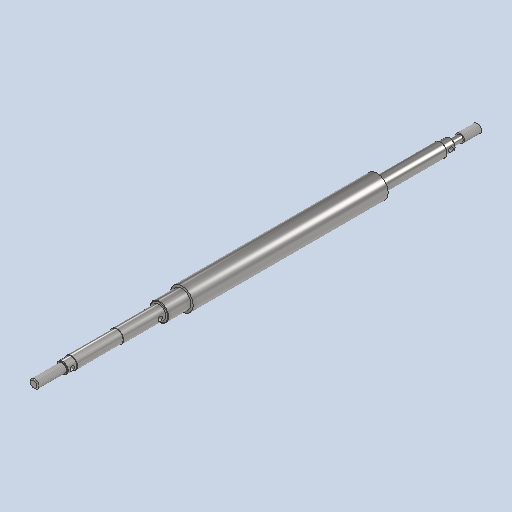
# Autodesk Inventor part: essieu arriere
Saved by Autodesk Inventor 2024 (Build 280153000, 153)
## iProperties
Created: 2022-10-04
Part Number: essieu arriere
Material: Acier inoxydable
Document SubType Name: Modeling
Designer: ropertth
Density: 8 g/cm^3
Appearance: Semi-poli
Mass: 74.8661 g
Surface Area: 48.0695 cm^2
Volume: 9.35827 cm^3
Author: ropertth
Autodesk Inventor part; units mm, degrees
ref_plane "YZ Plane" through (0, 0, 0) normal (1, 0, 0) x (0, 1, 0)
sketch "Esquisse1" plane through (0, 0, 0) normal (1, 0, 0) x (0, 1, 0)
  line L0 (5, -65) -> (5, -150.6)
  line L1 (5, -150.6) -> (2.9605, -150.6)
  line L2 (2.9605, -150.6) -> (2.9605, -178.6)
  line L3 (2.9605, -178.6) -> (1.919, -178.6)
  line L4 (1.919, -178.6) -> (1.919, -195.1)
  line L5 (1.919, -195.1) -> (0, -195.1)
  line L6 (4, -55) -> (2.9605, -55)
  line L7 (2.9605, -55) -> (2.9605, -36.5)
  line L8 (2.783, -16.5) -> (1.919, -16.5)
  line L9 (1.919, -16.5) -> (1.919, 0)
  line L10 (1.919, 0) -> (0, 0)
  line L11 (0, -195.1) -> (0, 0)
  line L12 (4, -55) -> (4, -65)
  line L13 (4, -65) -> (5, -65)
  line L14 (1.919, -16.5) -> (1.45, -16.5)
  line L15 (1.45, -16.5) -> (1.45, -8)
  line L16 (1.45, -8) -> (2, -8)
  line L17 (1.919, -12.5) -> (1.919, -16.5)
  line L18 (1.919, -178.6) -> (1.45, -178.6)
  line L19 (1.45, -178.6) -> (1.45, -187.1)
  line L20 (1.45, -187.1) -> (1.919, -187.1)
  line L21 (1.919, -187.1) -> (1.919, -178.6)
  line L22 (2.5, -16.5) -> (1.919, -16.5)
  line L23 (1.45, -12.5) -> (2.5, -12.5)
  line L24 (2.5, -12.5) -> (2.5, -16.5)
  line L25 (2.5, -178.6) -> (1.919, -178.6)
  line L26 (1.919, -178.6) -> (1.919, -182.6)
  line L27 (1.45, -182.6) -> (2.5, -182.6)
  line L28 (2.5, -182.6) -> (2.5, -178.6)
  line L29 (2.783, -16.5) -> (2.5, -16.5)
  line L30 (2.783, -16.5) -> (2.783, -36.5)
  line L31 (2.783, -36.5) -> (2.9605, -36.5)
  point P0 (1.919, -8)
  point P1 (1.919, -187.1)
  point P2 (2.4398, -178.6)
  point P3 (2.7415, -36.5)
  point P4 (2.7415, -16.5)
  dimension "d2" = 28
  dimension "d4" = 16.5
  dimension "d5" = 16.5
  dimension "d15" = 95.6
  dimension "d16" = 10
  dimension "d18" = 8.5
  dimension "d19" = 2.9
  dimension "d20" = 8.5
  dimension "d21" = 8
  dimension "d22" = 10
  dimension "d24" = 4
  dimension "d25" = 4
  dimension "d26" = 5
  dimension "d27" = 4
  dimension "d28" = 5
  dimension "d41" = 6
  constraints: 65 end point, 13 perpendicular, 9 point on line, 7 parallel, 6 horizontal, 2 collinear, 2 vertical, 1 midpoint
  measures "d2" distance of L1.end L2.end
  measures "d4" distance of L8.end L9.end
  measures "d5" distance of L3.end L4.end
  measures "d15" vertical distance of L0.end L6.end
  measures "d16" distance of L6.start L12.end
  measures "d18" distance of L14.end L15.end
  measures "d19" diameter of L15 L11
  measures "d20" distance of L18.end L19.end
  measures "d21" diameter of L12 L11
  measures "d22" diameter of L0 L11
  measures "d25" distance of L23.end L22.start
  measures "d26" diameter of L24 L11
  measures "d27" distance from line of point (2.44, -178.6) L27
  measures "d28" diameter of L28 L11
revolve "Révolution1" add sketch "Esquisse1" angle 360 about axis through (0, 0, -195.1) along (0, 0, 1) contours L0 L1 L2 L3 L18 L19 L20 L4 L5 L11 L10 L9 L16 L15 L14 L8 L30 L31 L7 L6 L12 L13 | L28 L27 L4 L3 | L4 L27 L19 L18 | L8 L9 L23 L24 | L14 L15 L23 L9 | L23 L15 L16 L9
fillet "Congé1" radius 0.5 2 edges at (0, -1.919, 0) (0, -1.919, -195.1)
thread "Filetage1" size "M4x0.7" class "6g" standard "ANSI Metric M Profile" full length
fillet "Congé2" radius 0.2 4 edges at (0, -2.5, -182.6) (0, -2.9605, -178.6) (0, -4, -55) (0, -2.5, -12.5)
sketch "Esquisse2" plane through (0, 0, -195.1) normal (0, 0, -1) x (-1, 0, 0)
  point P0 (0, 0)
  point P1 (0, 0)
  constraints: 1 coincident
hole "Perçage1" at (0, 0, -195.1) direction (0, 0, 1) diameter 1 depth 3 tip angle 118 countersink diameter 2 countersink angle 60
sketch "Esquisse3" plane through (0, 0, 0) normal (0, 0, 1) x (1, 0, 0)
  line L0 (0, 0) -> (-2.5, 0) construction
  circle A0 centre (0, 0) radius 2.5 construction
  circle A1 centre (0, 0) radius 2.5 construction
  line L1 (0, 0) -> (-5.0002, 0) construction
  circle A2 centre (0, 0) radius 2.9605 construction
  circle A3 centre (0, 0) radius 2.9605 construction
  point P0 (-2.9605, 0)
  constraints: 4 end point, 2 horizontal, 2 horizontal alignment, 1 coincident, 1 point on line, 2 other
ref_plane "Plan de construction1" through (-2.5, 0, 0) normal (-1, 0, 0) x (0, -1, 0)
sketch "Esquisse4" plane through (-2.5, 0, 0) normal (-1, 0, 0) x (0, -1, 0)
  line L0 (-4.9491, -12.5) -> (5.1773, -12.5)
  line L1 (5.1773, -12.5) -> (5.1773, -16.5)
  line L2 (5.1773, -16.5) -> (-4.9491, -16.5)
  line L3 (-4.9491, -16.5) -> (-4.9491, -12.5)
  line L4 (2.3, -182.6) -> (-2.3, -182.6) projected
  line L5 (2.7605, -178.6) -> (-2.7605, -178.6) projected
  line L6 (-3.4203, -182.6) -> (3.9321, -182.6)
  line L7 (3.9321, -182.6) -> (3.9321, -178.6)
  line L8 (3.9321, -178.6) -> (-3.4203, -178.6)
  line L9 (-3.4203, -178.6) -> (-3.4203, -182.6)
  point P0 (0, 0)
  constraints: 16 end point, 4 parallel, 2 horizontal, 2 perpendicular, 1 point on line
extrude "Extrusion1" cut sketch "Esquisse4" against normal blind 0.3
sketch "Esquisse6" plane through (-2.2, 0, 0) normal (-1, 0, 0) x (0, 0, 1)
  line L0 (0, 0) -> (-16.5, 0) construction
  line L1 (-16.5, 2.5) -> (-16.5, -2.5) construction
  line L2 (-12.5, 2.3) -> (-12.5, -2.3) construction
  line L3 (-178.6, -2.7605) -> (-178.6, 2.7605) projected
  line L4 (-182.6, -0.6708) -> (-182.6, 0.6708) projected
  point P0 (-14.5, 0)
  point P1 (-16.5, 1.1874)
  point P2 (-16.5, -1.1874)
  point P3 (-12.5, 0.6708)
  point P4 (-12.5, -0.6708)
  point P5 (-180.6, 0)
  dimension "d51" = 4
  dimension "d52" = 2
  dimension "d71" = 4
  dimension "d72" = 2
  constraints: 2 end point, 1 midpoint, 1 point on line
  measures "d51" distance between parallel lines of L1 L2
  measures "d52" distance from line of L2 point (-14.5, 0)
  measures "d71" distance between parallel lines of L3 L4
  measures "d72" distance from line of L3 point (-180.6, 0)
hole "Perçage2" at (-2.2, 0, -14.5) at (-2.2, 0, -180.6) direction (1, 0, 0) diameter 2 end through all
ref_plane "Plan de construction2" through (-2.9605, 0, 0) normal (-1, 0, 0) x (0, -1, 0)
sketch "Esquisse7" plane through (-2.9605, 0, 0) normal (-1, 0, 0) x (0, -1, 0)
  line L0 (-3.8, -55) -> (3.8, -55) construction
  line L1 (-5.1826, -55) -> (5.6831, -55)
  line L2 (5.6831, -55) -> (5.6831, -50.2)
  line L3 (5.6831, -50.2) -> (-5.1826, -50.2)
  line L4 (-5.1826, -50.2) -> (-5.1826, -55)
  point P0 (0, 0)
  dimension "d53" = 4.8
  constraints: 8 end point, 2 parallel, 1 collinear, 1 horizontal, 1 perpendicular
  measures "d53" distance between parallel lines of L3 L1
extrude "Extrusion2" cut sketch "Esquisse7" against normal blind 0.3
sketch "Esquisse8" plane through (-2.6605, 0, 0) normal (-1, 0, 0) x (0, 0, 1)
  line L0 (-55, -1.2986) -> (-55, 1.2986) projected
  point P0 (0, 0)
  point P1 (-52.6, 0)
  point P2 (-55, 0)
  dimension "d63" = 2.4
  constraints: 1 midpoint
  measures "d63" distance of point (-55, 0) point (-52.6, 0)
hole "Perçage4" at (-2.6605, 0, -52.6) direction (1, 0, 0) diameter 2 end through all
equation "\"d20\" = d18"
equation "\"d27\" = d25"
equation "\"d28\" = d26"
equation "\"d52\" = 0.5 * d51"
equation "\"d72\" = 0.5 * d71"
